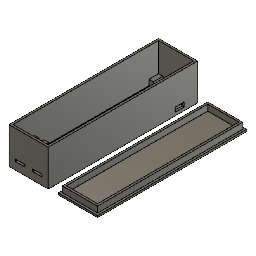
Moisture Stick Case (Autodesk Fusion 360 design; units mm, degrees)
Autodesk Fusion 360 part; units mm, degrees
sketch "Sketch1" plane through (0, 0, 0) normal (0, 1, 0) x (1, 0, 0)
  line L0 (0, 0) -> (26.1, 0)
  line L1 (26.1, 0) -> (26.1, 91.7)
  line L2 (26.1, 91.7) -> (0, 91.7)
  line L3 (0, 91.7) -> (0, 0)
  line L4 (3.175, 0) -> (22.925, 0)
  line L5 (22.925, 0) -> (22.925, -16)
  line L6 (22.925, -16) -> (3.175, -16)
  line L7 (3.175, -16) -> (3.175, 0)
  line L8 (10.3, -12) -> (15.8, -12)
  line L9 (15.8, -12) -> (15.8, -16)
  line L10 (15.8, -16) -> (10.3, -16)
  line L11 (10.3, -16) -> (10.3, -12)
  line L12 (0, 0) -> (26.1, 0)
  line L13 (26.1, 0) -> (26.1, -16)
  line L14 (26.1, -16) -> (0, -16)
  line L15 (0, -16) -> (0, 0)
  line L16 (-1.5, 93.2) -> (27.6, 93.2)
  line L17 (27.6, 93.2) -> (27.6, -17.5)
  line L18 (27.6, -17.5) -> (-1.5, -17.5)
  line L19 (-1.5, -17.5) -> (-1.5, 93.2)
  line L20 (0, 91.7) -> (3.3, 91.7)
  line L21 (3.3, 91.7) -> (3.3, 84.7)
  line L22 (3.3, 84.7) -> (0, 84.7)
  line L23 (0, 84.7) -> (0, 91.7)
  line L24 (26.1, 84.7) -> (22.8, 84.7)
  line L25 (22.8, 91.7) -> (26.1, 91.7)
  line L26 (26.1, 91.7) -> (26.1, 84.7)
  line L27 (22.8, 84.7) -> (22.8, 91.7)
  line L28 (3.3, 0) -> (0, 0)
  line L29 (0, 7) -> (3.3, 7)
  line L30 (3.3, 7) -> (3.3, 0)
  line L31 (0, 0) -> (0, 7)
  line L32 (26.1, 0) -> (22.8, 0)
  line L33 (22.8, 7) -> (26.1, 7)
  line L34 (26.1, 7) -> (26.1, 0)
  line L35 (22.8, 0) -> (22.8, 7)
  line L36 (3.175, 0) -> (8.175, 0)
  line L37 (8.175, 0) -> (8.175, -16)
  line L38 (8.175, -16) -> (3.175, -16)
  line L39 (3.175, -16) -> (3.175, 0)
  line L40 (17.925, 0) -> (22.925, 0)
  line L41 (22.925, 0) -> (22.925, -16)
  line L42 (22.925, -16) -> (17.925, -16)
  line L43 (17.925, -16) -> (17.925, 0)
  dimension "d1" = 91.7
  dimension "d2" = 26.1
  dimension "d3" = 16
  dimension "d4" = 19.75
  dimension "d5" = 5.5
  dimension "d6" = 4
  dimension "d7" = 1.5
  dimension "d8" = 1.5
  dimension "d9" = 1.5
  dimension "d10" = 1.5
  dimension "d15" = 3.3
  dimension "d16" = 7
  dimension "d17" = 3.3
  dimension "d18" = 7
  dimension "d19" = 3.3
  dimension "d20" = 7
  dimension "d21" = 3.3
  dimension "d22" = 7
  dimension "d29" = 5
  dimension "d30" = 5
  constraint horizontal L0
  constraint vertical L1
  constraint horizontal L2
  constraint vertical L3
  constraint coincident L0.start L3.end
  constraint horizontal L4
  constraint vertical L5
  constraint horizontal L6
  constraint vertical L7
  constraint horizontal L8
  constraint vertical L9
  constraint horizontal L10
  constraint vertical L11
  constraint midpoint L0 L4
  constraint collinear L6 L10
  constraint midpoint L6 L10
  constraint horizontal L12
  constraint vertical L13
  constraint horizontal L14
  constraint vertical L15
  constraint collinear L6 L14
  constraint horizontal L16
  constraint vertical L17
  constraint horizontal L18
  constraint vertical L19
  constraint horizontal L20
  constraint vertical L21
  constraint horizontal L22
  constraint vertical L23
  constraint horizontal L25
  constraint vertical L26
  constraint horizontal L24
  constraint vertical L27
  constraint horizontal L29
  constraint vertical L30
  constraint horizontal L28
  constraint vertical L31
  constraint horizontal L33
  constraint vertical L34
  constraint horizontal L32
  constraint vertical L35
  constraint collinear L2 L20
  constraint collinear L3 L23
  constraint collinear L2 L25
  constraint collinear L1 L26
  constraint collinear L0 L28
  constraint collinear L3 L31
  constraint collinear L0 L32
  constraint collinear L1 L34
  constraint horizontal L36
  constraint vertical L37
  constraint horizontal L38
  constraint vertical L39
  constraint collinear L4 L36
  constraint collinear L6 L38
  constraint collinear L7 L39
  constraint horizontal L40
  constraint vertical L41
  constraint horizontal L42
  constraint vertical L43
  constraint collinear L4 L40
  constraint collinear L6 L42
  constraint collinear L5 L41
  measures "d1" distance of L0.start L2.end
  measures "d2" distance of L1.end L2.end
  measures "d3" distance of L4.start L6.end
  measures "d4" distance of L4.start L4.end
  measures "d5" distance of L8.start L8.end
  measures "d6" distance of L8.start L10.end
  measures "d7" distance of L2 L16
  measures "d8" distance of L3 L19
  measures "d9" distance of L1 L17
  measures "d10" distance of L14 L18
  measures "d15" distance of L2.end L20.end
  measures "d16" distance of L2.end L22.end
  measures "d17" distance of L1.end L25.start
  measures "d18" distance of L24.end L25.start
  measures "d19" distance of L29.end L29.start
  measures "d20" distance of L0.start L29.start
  measures "d21" distance of L33.end L33.start
  measures "d22" distance of L32.end L33.start
  measures "d29" distance of L4.start L36.end
  measures "d30" distance of L40.start L4.end
extrude "Extrude1" add sketch "Sketch1" along normal blind 27 makes body 1
extrude "Extrude2" add sketch "Sketch1" along normal blind 1.5 contours L0 L3 L4 L12 L28 L29 L30 L31 L36 | L0 L7 L12 L14 L15 L28 L39 | L0 L4 L6 L7 L12 L14 L28 L36 L37 L38 L39 | L0 L1 L2 L3 L4 L12 L21 L22 L24 L27 L29 L30 L33 L35 L36 L40 | L2 L3 L20 L21 L22 L23 | L0 L4 L6 L8 L9 L11 L12 L14 L37 L43 | L0 L4 L5 L6 L12 L14 L32 L40 L41 L42 L43 | L6 L8 L9 L10 L11 L14 | L0 L1 L4 L12 L32 L33 L34 L35 L40 | L1 L2 L24 L25 L26 L27 | L0 L5 L12 L13 L14 L32 L41 bodies 1
extrude "Extrude3" add sketch "Sketch1" along normal blind 5.7 contours L0 L3 L4 L12 L28 L29 L30 L31 L36 | L2 L3 L20 L21 L22 L23 | L0 L1 L4 L12 L32 L33 L34 L35 L40 | L1 L2 L24 L25 L26 L27 bodies 1
extrude "Extrude4" add sketch "Sketch1" along normal blind 12 contours L0 L7 L12 L14 L15 L28 L39 | L6 L8 L9 L10 L11 L14 | L0 L5 L12 L13 L14 L32 L41 bodies 1
fillet "Fillet1" radius 2.75 2 edges at (15.8, 6.75, 12) (10.3, 6.75, 12) on bodies 1
extrude "Extrude5" add sketch "Sketch1" along normal blind 5.7 contours L0 L4 L6 L7 L12 L14 L28 L36 L37 L38 L39 | L0 L4 L5 L6 L12 L14 L32 L40 L41 L42 L43 bodies 1
sketch "Sketch2" plane through (0, 0, 17.5) normal (0, 0, 1) x (1, 0, 0)
  line L0 (-1.5, 0) -> (27.6, 0)
  line L1 (27.6, 0) -> (27.6, 27)
  line L2 (27.6, 27) -> (-1.5, 27)
  line L3 (-1.5, 27) -> (-1.5, 0)
  line L4 (3.175, 5.7) -> (10.175, 5.7)
  line L5 (10.175, 5.7) -> (10.175, 7.3)
  line L6 (10.175, 7.3) -> (3.175, 7.3)
  line L7 (3.175, 7.3) -> (3.175, 5.7)
  line L8 (0, 5.7) -> (0, 1.5)
  line L9 (27.6, 0) -> (-1.5, 0)
  line L10 (15.925, 7.3) -> (22.925, 7.3)
  line L11 (22.925, 7.3) -> (22.925, 5.7)
  line L12 (22.925, 5.7) -> (15.925, 5.7)
  line L13 (15.925, 5.7) -> (15.925, 7.3)
  dimension "d33" = 5.7
  dimension "d34" = 4.675
  dimension "d35" = 7
  dimension "d36" = 1.6
  dimension "d37" = 1.6
  dimension "d38" = 7
  dimension "d39" = 4.675
  dimension "d40" = 5.7
  constraint horizontal L4
  constraint vertical L5
  constraint horizontal L6
  constraint vertical L7
  constraint horizontal L10
  constraint vertical L11
  constraint horizontal L12
  constraint vertical L13
  measures "d33" distance of L4 L9
  measures "d34" distance of L3 L7
  measures "d35" distance of L5.end L6.end
  measures "d36" distance of L4.end L5.end
  measures "d37" distance of L10.start L12.end
  measures "d38" distance of L10.start L10.end
  measures "d39" distance of L1 L11
  measures "d40" distance of L9 L12
extrude "Extrude6" cut sketch "Sketch2" against normal blind 4 contours L4 L5 L6 L7 | L10 L11 L12 L13 bodies 1
sketch "Sketch3" plane through (27.6, 0, 0) normal (1, 0, 0) x (0, 0, -1)
  line L0 (-17.5, 0) -> (93.2, 0)
  line L1 (93.2, 0) -> (93.2, 27)
  line L2 (93.2, 27) -> (-17.5, 27)
  line L3 (-17.5, 27) -> (-17.5, 0)
  line L4 (76.6, 2.4) -> (83.2, 2.4)
  line L5 (83.2, 2.4) -> (83.2, 5.7)
  line L6 (83.2, 5.7) -> (76.6, 5.7)
  line L7 (76.6, 5.7) -> (76.6, 2.4)
  line L8 (93.2, 0) -> (-17.5, 0)
  dimension "d43" = 6.6
  dimension "d44" = 3.3
  dimension "d45" = 10
  dimension "d46" = 2.4
  constraint horizontal L4
  constraint vertical L5
  constraint horizontal L6
  constraint vertical L7
  measures "d43" distance of L5.end L6.end
  measures "d44" distance of L4.start L6.end
  measures "d45" distance of L1 L5
  measures "d46" distance of L4 L8
extrude "Extrude7" cut sketch "Sketch3" against normal blind 4 contours L4 L5 L6 L7 bodies 1
sketch "Sketch4" plane through (0, 0, 0) normal (0, 1, 0) x (1, 0, 0)
  line L0 (0, 0) -> (29.1, 0)
  line L1 (29.1, 0) -> (29.1, 110.7)
  line L2 (29.1, 110.7) -> (0, 110.7)
  line L3 (0, 110.7) -> (0, 0)
  line L4 (1.5, 109.2) -> (27.6, 109.2)
  line L5 (27.6, 109.2) -> (27.6, 1.5)
  line L6 (27.6, 1.5) -> (1.5, 1.5)
  line L7 (1.5, 1.5) -> (1.5, 109.2)
  line L8 (3, 107.7) -> (26.1, 107.7)
  line L9 (26.1, 107.7) -> (26.1, 3)
  line L10 (26.1, 3) -> (3, 3)
  line L11 (3, 3) -> (3, 107.7)
  dimension "d49" = 110.7
  dimension "d50" = 29.1
  dimension "d51" = 1.5
  dimension "d52" = 1.5
  dimension "d53" = 1.5
  dimension "d54" = 1.5
  dimension "d55" = 1.5
  dimension "d56" = 1.5
  dimension "d57" = 1.5
  dimension "d58" = 1.5
  constraint horizontal L0
  constraint vertical L1
  constraint horizontal L2
  constraint vertical L3
  constraint coincident L0.start L3.end
  constraint horizontal L4
  constraint vertical L5
  constraint horizontal L6
  constraint vertical L7
  constraint horizontal L8
  constraint vertical L9
  constraint horizontal L10
  constraint vertical L11
  measures "d49" distance of L0.start L2.end
  measures "d50" distance of L0.start L0.end
  measures "d51" distance of L2 L4
  measures "d52" distance of L3 L7
  measures "d53" distance of L1 L5
  measures "d54" distance of L0 L6
  measures "d55" distance of L4 L8
  measures "d56" distance of L7 L11
  measures "d57" distance of L5 L9
  measures "d58" distance of L6 L10
extrude "Extrude8" add sketch "Sketch4" along normal blind 1.5 separate body contours L0 L1 L2 L3 | L4 L5 L6 L7 | L8 L9 L10 L11 makes body 2
extrude "Extrude9" add sketch "Sketch4" along normal blind 6 contours L4 L5 L6 L7 bodies 2
move_body "Move1" bodies 2 to x (1, 0, 0) y (0, 1, 0) z (0, 0, 1) at (35, 0, 17.5)
